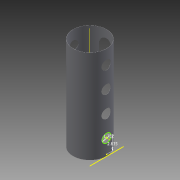
# Autodesk Inventor part: Probe Region Shield
Saved by Autodesk Inventor 2015 (Build 190159000, 159)
## iProperties
Created: 2014-06-23
Part Number: Probe Region Shield
Material: Generic
Document SubType Name: Modeling
Designer: Aki
Density: 1 g/cm^3
Appearance: Default
Author: Aki
Autodesk Inventor part; units mm, degrees
ref_plane "XZ Plane" through (0, 0, 0) normal (0, 1, 0) x (-1, 0, 0)
sketch "Sketch1" plane through (0, 0, 0) normal (0, 1, 0) x (-1, 0, 0)
  circle A0 centre (0, 0) radius 84.5
  circle A1 centre (0, 0) radius 85.5
  dimension "d0" = 169
  dimension "d1" = 171
  constraints: 2 centre point, 2 coincident
  measures "d0" diameter of A0
  measures "d1" diameter of A1
extrude "Extrusion1" add sketch "Sketch1" along normal blind 466.5 and the other way blind 7.989
ref_plane "Work Plane1" through (85.5, 0, 0) normal (1, 0, 0) x (0, 1, 0)
ref_plane "Work Plane2" through (-85.5, 0, 0) normal (1, 0, 0) x (0, 1, 0)
sketch "Sketch2" plane through (85.5, 0, 0) normal (1, 0, 0) x (0, 1, 0)
  circle A0 centre (394.5, 0) radius 23.25
  line L0 (466.5, -85.5) -> (466.5, 85.5) projected
  line L1 (-7.989, 85.5) -> (-7.989, -85.5) projected
  point P0 (0, 0)
  dimension "d9" = 46.5
  dimension "d12" = 72
  constraints: 1 centre point, 1 other
  measures "d9" diameter of A0
  measures "d12" distance from line of L0 A0.centre
hole "Hole1" at (85.5, 394.5, 0) direction (-1, 0, 0) diameter 46.5 end through all
sketch "Sketch3" plane through (85.5, 0, 0) normal (1, 0, 0) x (0, 1, 0)
  circle A0 centre (72, 0) radius 23.25
  line L0 (-7.989, 85.5) -> (-7.989, -85.5) projected
  point P0 (0, 0)
  dimension "d21" = 46.5
  dimension "d60" = 72
  constraints: 1 centre point, 1 other
  measures "d21" diameter of A0
  measures "d60" distance of A0.centre point (0, 0)
hole "Hole2" at (85.5, 72, 0) direction (-1, 0, 0) diameter 46.5 end through all
sketch "Sketch4" plane through (85.5, 0, 0) normal (1, 0, 0) x (0, 1, 0)
  circle A0 centre (179.5, 0) radius 23.25
  line L0 (-7.989, 85.5) -> (-7.989, -85.5) projected
  point P0 (0, 0)
  dimension "d30" = 46.5
  dimension "d61" = 179.5
  constraints: 1 centre point, 1 other
  measures "d30" diameter of A0
  measures "d61" distance of A0.centre point (0, 0)
hole "Hole3" at (85.5, 179.5, 0) direction (-1, 0, 0) diameter 46.5 end through all
sketch "Sketch5" plane through (85.5, 0, 0) normal (1, 0, 0) x (0, 1, 0)
  circle A0 centre (287, 0) radius 23.25
  line L0 (-7.989, 85.5) -> (-7.989, -85.5) projected
  point P0 (0, 0)
  dimension "d39" = 46.5
  dimension "d62" = 287
  constraints: 1 centre point, 1 other
  measures "d39" diameter of A0
  measures "d62" distance of A0.centre point (0, 0)
hole "Hole4" at (85.5, 287, 0) direction (-1, 0, 0) diameter 46.5 end through all
sketch "Sketch6" plane through (85.5, 0, 0) normal (1, 0, 0) x (0, 1, 0)
  circle A0 centre (72, 0) radius 22.25
  line L0 (-7.989, 85.5) -> (-7.989, -85.5) projected
  point P0 (0, 0)
  dimension "d48" = 44.5
  dimension "d63" = 72
  constraints: 1 centre point, 1 other
  measures "d48" diameter of A0
  measures "d63" distance of point (0, 0) A0.centre
ref_plane "Work Plane4" through (0, 0, -85.5) normal (0, 0, 1) x (1, 0, 0)
sketch "Sketch9" plane through (0, 0, -85.5) normal (0, 0, 1) x (1, 0, 0)
  circle A0 centre (0, 394.5) radius 32.75
  line L0 (85.5, 466.5) -> (-85.5, 466.5) projected
  line L1 (-85.5, -7.989) -> (85.5, -7.989) projected
  line L2 (32.75, 394.5) -> (-32.75, 394.5)
  line L3 (-32.75, 394.5) -> (-32.75, -7.989)
  line L4 (-32.75, -7.989) -> (32.75, -7.989)
  line L5 (32.75, -7.989) -> (32.75, 394.5)
  point P0 (0, 0)
  dimension "d51" = 65.5
  dimension "d52" = 72
  dimension "d53" = 65.5
  dimension "d56" = 0
  dimension "d57" = 0
  constraints: 8 end point, 2 parallel, 1 horizontal, 1 horizontal alignment, 1 perpendicular, 4 other
  measures "d52" distance from line of point (0, 394.5) L0
  measures "d53" distance of L4.end L3.end
  measures "d56" horizontal distance of point (0, 0) point (0, 394.5)
  measures "d57" distance from line of point (0, 394.5) L2
extrude "Extrusion2" cut sketch "Sketch9" along normal blind 25.4
body "Solid1"
